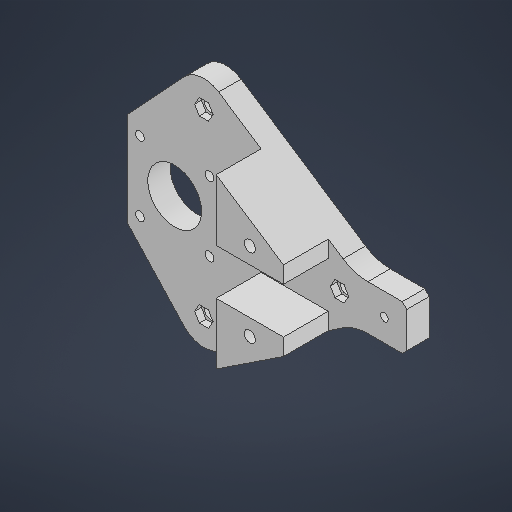
# Autodesk Inventor part: y axis motor holder
Saved by Autodesk Inventor 2025.1 (Build 291241000, 241)
## iProperties
Created: 2025-02-02
Part Number: y axis motor holder
Material: Generic
Document SubType Name: Modeling
Designer: jerem
Density: 1 g/cm^3
Appearance: Default
Author: jerem
## iProperties of the stored document y axis motor holder_3DPrint.ipt
Created: 2025-02-21
Part Number: y axis motor holder_3DPrint
Material: Generic
Document SubType Name: Modeling
Designer: jerem
Density: 1 g/cm^3
Appearance: Default
Author: jerem
Autodesk Inventor part; units mm, degrees
ref_plane "YZ Plane" through (0, 0, 0) normal (1, 0, 0) x (0, 1, 0)
ref_plane "XZ Plane" through (0, 0, 0) normal (0, 1, 0) x (-1, 0, 0)
ref_plane "XY Plane" through (0, 0, 0) normal (0, 0, 1) x (1, 0, 0)
sketch "Sketch1" plane through (0, 0, 0) normal (0, 0, 1) x (1, 0, 0)
  line L0 (0, 0) -> (30.25, 0) construction
  line L1 (0, 0) -> (-30.25, 0) construction
  line L2 (-30.25, 0) -> (-30.25, 40) construction
  line L3 (-30.25, 0) -> (-30.25, -40) construction
  circle A0 centre (-30.25, 40) radius 2.7
  circle A1 centre (-30.25, -40) radius 2.7
  circle A2 centre (30.25, 0) radius 2.7
  circle A3 centre (-30.25, 40) radius 12
  circle A4 centre (-30.25, -40) radius 12
  circle A5 centre (30.25, 0) radius 12
  line L4 (36.8682, -10.01) -> (-23.6318, -50.01)
  line L5 (-42.25, 40) -> (-42.25, -40)
  line L6 (-23.6318, 50.01) -> (36.8682, 10.01)
  line L7 (30.25, 0) -> (50.25, 0) construction
  circle A6 centre (50.25, 0) radius 10
  circle A7 centre (50.25, 0) radius 1.75
  line L8 (50.2575, 10) -> (36.8682, 10.01)
  line L9 (50.2575, -10) -> (36.8682, -10.01)
  line L10 (-27.75, -15.5) -> (-58.75, -15.5) construction
  line L11 (-58.75, -15.5) -> (-58.75, 15.5) construction
  line L12 (-58.75, 15.5) -> (-27.75, 15.5) construction
  line L13 (-27.75, 15.5) -> (-27.75, -15.5) construction
  line L14 (-27.75, -15.5) -> (-58.75, 15.5) construction
  line L15 (-58.75, -15.5) -> (-27.75, 15.5) construction
  line L16 (-22.25, -21) -> (-64.25, -21) construction
  line L17 (-64.25, -21) -> (-64.25, 21)
  line L18 (-64.25, 21) -> (-22.25, 21) construction
  line L19 (-22.25, 21) -> (-22.25, -21) construction
  line L20 (-22.25, -21) -> (-64.25, 21) construction
  line L21 (-64.25, -21) -> (-22.25, 21) construction
  line L22 (-43.25, 0) -> (-42.25, 0) construction
  circle A8 centre (-27.75, 15.5) radius 2
  circle A9 centre (-58.75, 15.5) radius 2
  circle A10 centre (-58.75, -15.5) radius 2
  circle A11 centre (-27.75, -15.5) radius 2
  line L23 (-64.25, 21) -> (-39.0465, 48.1622)
  line L24 (-64.25, -21) -> (-39.0465, -48.1622)
  circle A12 centre (-43.25, 0) radius 12
  circle A13 centre (10.25, 0) radius 1.75
  line L25 (50.2575, 10) -> (60.2575, 9.9925)
  line L26 (60.2575, 9.9925) -> (60.2425, -9.9925)
  line L27 (60.2425, -9.9925) -> (50.2575, -10)
  point P0 (41.35, -4.5596)
  point P1 (41.35, 4.5596)
  point P2 (60.25, -0.0075)
  dimension "d0" = 60.5
  dimension "d1" = 5.4
  dimension "d2" = 80
  dimension "d3" = 24
  dimension "d57" = 20
  dimension "d58" = 20
  dimension "d61" = 31
  dimension "d63" = 42
  dimension "d65" = 1
  dimension "d66" = 4
  dimension "d67" = 4
  dimension "d68" = 4
  dimension "d69" = 4
  dimension "d70" = 3.5
  dimension "d71" = 24
  dimension "d74" = 3.5
  dimension "d75" = 20
  constraints: 56 end point, 14 centre point, 13 coincident, 12 tangent, 10 point on circle, 6 horizontal, 5 midpoint, 4 equal length, 4 equal radius, 4 parallel, 4 perpendicular, 2 point on line, 2 vertical, 1 collinear
  measures "d0" distance of L0.end L1.end
  measures "d1" diameter of A0
  measures "d2" distance of L3.end L2.end
  measures "d3" diameter of A3
  measures "d57" distance of L7.start L7.end
  measures "d58" diameter of A6
  measures "d61" distance of L10.end L11.end
  measures "d63" distance of L16.end L17.end
  measures "d65" distance of L22.end L22.start
  measures "d66" diameter of A8
  measures "d67" diameter of A9
  measures "d68" diameter of A10
  measures "d69" diameter of A11
  measures "d70" diameter of A7
  measures "d71" diameter of A12
  measures "d74" diameter of A13
  measures "d75" distance of L0.end A13.centre
extrude "Extrusion1" add sketch "Sketch1" against normal blind 10 contours A3 | A3 L6 A5 L4 A4 L5 A12 | L26 L27 A6 | L5 A12 A4 L24 L17 L23 A3 | A5 A6 | L8 A6 A5 | A5 A6 L9 | A6 A5 | A5 A6 | L25 L26 A6 | A4
fillet "Fillet1" radius 20 2 edges at (36.8682, 10.01, -5) (36.8682, -10.01, -5)
chamfer "Chamfer7" distance 2 angle 45 2 edges at (60.2575, 9.9925, -5) (60.2425, -9.9925, -5)
sketch "Sketch8" plane through (0, 0, 0) normal (0, 0, 1) x (1, 0, 0)
  line L0 (58.2425, -9.994) -> (60.244, -7.9925) projected
  line L1 (58.2425, -9.994) -> (42.8738, -10.0055) projected
  arc A0 (42.8738, -10.0055) -> (31.8585, -13.3222) centre (42.8887, -30.0055) ccw projected
  line L2 (31.8585, -13.3222) -> (-23.6318, -50.01) projected
  arc A1 (-39.0465, -48.1622) -> (-23.6318, -50.01) centre (-30.25, -40) ccw projected
  line L3 (-39.0465, -48.1622) -> (-64.25, -21) projected
  line L4 (-64.25, -21) -> (-64.25, 21) projected
  line L5 (-64.25, 21) -> (-39.0465, 48.1622) projected
  arc A2 (-23.6318, 50.01) -> (-39.0465, 48.1622) centre (-30.25, 40) ccw projected
  line L6 (-23.6318, 50.01) -> (31.8585, 13.3222) projected
  arc A3 (31.8585, 13.3222) -> (42.8738, 10.0055) centre (42.8887, 30.0055) ccw projected
  line L7 (42.8738, 10.0055) -> (58.2575, 9.994) projected
  line L8 (60.256, 7.9925) -> (58.2575, 9.994) projected
  line L9 (60.256, 7.9925) -> (60.244, -7.9925) projected
  circle A4 centre (30.25, 0) radius 2.7 projected
  circle A5 centre (50.25, 0) radius 1.75 projected
  circle A6 centre (-30.25, -40) radius 2.7 projected
  circle A7 centre (-43.25, 0) radius 12 projected
  circle A8 centre (-58.75, -15.5) radius 2 projected
  circle A9 centre (-58.75, 15.5) radius 2 projected
  circle A10 centre (10.25, 0) radius 1.75 projected
  circle A11 centre (-27.75, 15.5) radius 2 projected
  circle A12 centre (-27.75, -15.5) radius 2 projected
  circle A13 centre (-30.25, 40) radius 2.7 projected
  line L10 (-32.2996, 43.55) -> (-28.2004, 43.55)
  line L11 (-28.2004, 43.55) -> (-26.1508, 40)
  line L12 (-26.1508, 40) -> (-28.2004, 36.45)
  line L13 (-28.2004, 36.45) -> (-32.2996, 36.45)
  line L14 (-32.2996, 36.45) -> (-34.3492, 40)
  line L15 (-34.3492, 40) -> (-32.2996, 43.55)
  line L16 (28.2004, 3.55) -> (32.2996, 3.55)
  line L17 (32.2996, 3.55) -> (34.3492, 0)
  line L18 (34.3492, 0) -> (32.2996, -3.55)
  line L19 (32.2996, -3.55) -> (28.2004, -3.55)
  line L20 (28.2004, -3.55) -> (26.1508, 0)
  line L21 (26.1508, 0) -> (28.2004, 3.55)
  line L22 (-32.2996, -36.45) -> (-28.2004, -36.45)
  line L23 (-28.2004, -36.45) -> (-26.1508, -40)
  line L24 (-26.1508, -40) -> (-28.2004, -43.55)
  line L25 (-28.2004, -43.55) -> (-32.2996, -43.55)
  line L26 (-32.2996, -43.55) -> (-34.3492, -40)
  line L27 (-34.3492, -40) -> (-32.2996, -36.45)
  point P0 (0, 0)
  dimension "d97" = 7.1
  dimension "d98" = 7.1
  dimension "d99" = 7.1
  constraints: 36 end point, 3 coincident, 3 horizontal, 39 other
  measures "d97" distance between parallel lines of L13 L10
  measures "d98" distance between parallel lines of L19 L16
  measures "d99" distance between parallel lines of L25 L22
extrude "Extrusion9" cut sketch "Sketch8" against normal blind 3 contours L10 L11 L12 L13 L14 L15 | L16 L17 L18 L19 L20 L21 | L22 L23 L24 L25 L26 L27
sketch "Sketch5" plane through (0, 0, 0) normal (0, 0, 1) x (1, 0, 0)
  line L0 (42.8738, -10.0055) -> (58.2425, -9.994) projected
  arc A0 (31.8585, 13.3222) -> (42.8738, 10.0055) centre (42.8887, 30.0055) ccw projected
  line L1 (31.8585, 13.3222) -> (-23.6318, 50.01) projected
  arc A1 (-23.6318, 50.01) -> (-39.0465, 48.1622) centre (-30.25, 40) ccw projected
  line L2 (-39.0465, 48.1622) -> (-64.25, 21) projected
  line L3 (-64.25, 21) -> (-64.25, -21) projected
  line L4 (-64.25, -21) -> (-39.0465, -48.1622) projected
  arc A2 (-39.0465, -48.1622) -> (-23.6318, -50.01) centre (-30.25, -40) ccw projected
  line L5 (-23.6318, -50.01) -> (31.8585, -13.3222) projected
  arc A3 (42.8738, -10.0055) -> (31.8585, -13.3222) centre (42.8887, -30.0055) ccw projected
  circle A4 centre (50.25, 0) radius 1.75 projected
  circle A5 centre (-27.75, -15.5) radius 2 projected
  circle A6 centre (-27.75, 15.5) radius 2 projected
  circle A7 centre (-58.75, 15.5) radius 2 projected
  circle A8 centre (-58.75, -15.5) radius 2 projected
  circle A9 centre (-43.25, 0) radius 12 projected
  line L6 (-4.75, -10.2) -> (-4.75, -37.5261)
  line L7 (25.25, -10.2) -> (25.25, -17.6914)
  line L8 (-4.75, -10.2) -> (25.25, -10.2)
  line L9 (60.244, -7.9925) -> (60.256, 7.9925) projected
  line L10 (58.2575, 9.994) -> (42.8738, 10.0055) projected
  line L11 (60.244, -7.9925) -> (58.2425, -9.994) projected
  line L12 (58.2575, 9.994) -> (60.256, 7.9925) projected
  point P0 (0, 0)
  dimension "d92" = 30
  dimension "d93" = 10.2
  dimension "d106" = 25
  constraints: 6 end point, 2 point on line, 1 horizontal, 1 parallel, 1 vertical
  measures "d92" distance of L6.start L7.start
  measures "d93" distance from line of L8 point (0, 0)
  measures "d106" distance from line of A4.centre L7
extrude "Extrusion6" add sketch "Sketch5" along normal blind 20 contours L5 L6 L8 L7
sketch "Sketch9" plane through (0, 0, 20) normal (0, 0, 1) x (1, 0, 0)
  circle A0 centre (10.25, 0) radius 1.75 projected
  line L0 (-4.75, -10.2) -> (-4.75, -37.5261) projected
  line L1 (-4.75, -37.5261) -> (25.25, -17.6914) projected
  line L2 (25.25, -17.6914) -> (25.25, -10.2) projected
  line L3 (25.25, -10.2) -> (-4.75, -10.2) projected
  line L4 (10.25, 0) -> (10.25, -17.5) construction
  circle A1 centre (10.25, -17.5) radius 2.5
  point P0 (0, 0)
  dimension "d102" = 17.5
  dimension "d103" = 5
  constraints: 2 end point, 1 centre point, 1 coincident, 1 vertical
  measures "d102" distance of L4.start L4.end
  measures "d103" diameter of A1
extrude "Extrusion10" cut sketch "Sketch9" against normal blind 5 contours A1
mirror "Mirror1" about plane through (0, 0, 0) normal (0, 1, 0) of "Extrusion6", "Extrusion10"
equation "\"b\" = 2"
body "Solid1"
